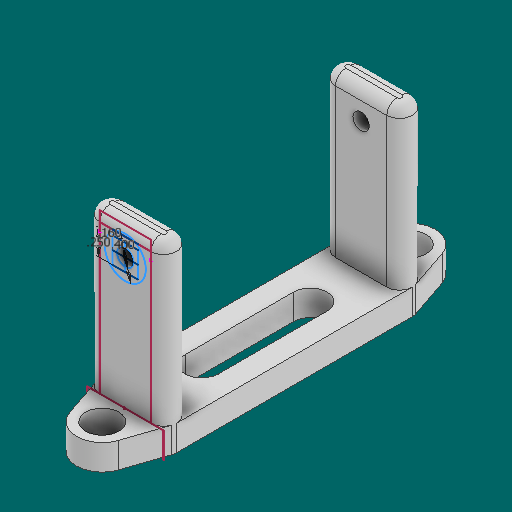
# Autodesk Inventor part: Latest_Odom
Saved by Autodesk Inventor 2025.2 (Build 292293000, 293)
## iProperties
Created: 2024-11-18
Part Number: Latest_Odom
Material: Generic
Document SubType Name: Modeling
Designer: colli
Density: 1 g/cm^3
Appearance: Default
Author: colli
Autodesk Inventor part; units mm, degrees
ref_plane "YZ Plane" through (0, 0, 0) normal (1, 0, 0) x (0, 1, 0)
ref_plane "XZ Plane" through (0, 0, 0) normal (0, 1, 0) x (-1, 0, 0)
ref_plane "XY Plane" through (0, 0, 0) normal (0, 0, 1) x (1, 0, 0)
sketch "Sketch1" plane through (0, 0, 0) normal (0, 1, 0) x (-1, 0, 0)
  line L0 (1.8331, -34.925) -> (-1.8331, -34.925)
  line L1 (-1.8331, -34.925) -> (-3.6662, -31.75)
  line L2 (-3.6662, -31.75) -> (-1.8331, -28.575)
  line L3 (-1.8331, -28.575) -> (1.8331, -28.575)
  line L4 (1.8331, -28.575) -> (3.6662, -31.75)
  line L5 (3.6662, -31.75) -> (1.8331, -34.925)
  circle A0 centre (0, -31.75) radius 2.0955
  circle A1 centre (0, -31.75) radius 3.0353
  line L6 (-31.877, 19.812) -> (-31.877, -7.112)
  line L7 (-31.877, -7.112) -> (31.877, -7.112)
  line L8 (31.877, -7.112) -> (31.877, 19.812)
  line L9 (31.877, 19.812) -> (-31.877, 19.812)
  line L10 (0, 6.35) -> (31.877, 6.35)
  line L11 (0, 6.35) -> (-31.877, 6.35)
  arc A2 (-6.0168, -33.7799) -> (6.0168, -33.7799) centre (0, -31.75) ccw
  line L12 (-6.35, -26.035) -> (6.35, -26.035)
  line L13 (6.35, -19.685) -> (-6.35, -19.685)
  arc A3 (-6.35, -19.685) -> (-6.35, -26.035) centre (-6.35, -22.86) ccw
  arc A4 (6.35, -26.035) -> (6.35, -19.685) centre (6.35, -22.86) ccw
  line L14 (9.525, -22.86) -> (9.525, -7.112)
  line L15 (6.0168, -33.7799) -> (9.3584, -23.8749)
  line L16 (-9.525, -7.112) -> (-9.525, -22.86)
  line L17 (-9.3584, -23.8749) -> (-6.0168, -33.7799)
  line L18 (1.8331, 47.625) -> (-1.8331, 47.625)
  line L19 (-1.8331, 47.625) -> (-3.6662, 44.45)
  line L20 (-3.6662, 44.45) -> (-1.8331, 41.275)
  line L21 (-1.8331, 41.275) -> (1.8331, 41.275)
  line L22 (1.8331, 41.275) -> (3.6662, 44.45)
  line L23 (3.6662, 44.45) -> (1.8331, 47.625)
  circle A5 centre (0, 44.45) radius 2.0955
  circle A6 centre (0, 44.45) radius 3.0353
  arc A7 (6.0168, 46.4799) -> (-6.0168, 46.4799) centre (0, 44.45) ccw
  line L24 (-6.35, 38.735) -> (6.35, 38.735)
  line L25 (6.35, 32.385) -> (-6.35, 32.385)
  arc A8 (-6.35, 38.735) -> (-6.35, 32.385) centre (-6.35, 35.56) ccw
  arc A9 (6.35, 32.385) -> (6.35, 38.735) centre (6.35, 35.56) ccw
  line L26 (6.0168, 46.4799) -> (9.3584, 36.5749)
  line L27 (-9.3584, 36.5749) -> (-6.0168, 46.4799)
  line L28 (9.525, 35.56) -> (9.525, 19.812)
  line L29 (-9.525, 35.56) -> (-9.525, 19.812)
  circle A10 centre (0, 44.45) radius 4.1275
  circle A11 centre (0, -31.75) radius 4.1275
  line L30 (-9.525, 19.812) -> (-9.525, -7.112)
  line L31 (9.525, 19.812) -> (9.525, -7.112)
  line L32 (0, 19.812) -> (0, -7.112) construction
  line L33 (4.1275, 19.812) -> (4.1275, -7.112)
  line L34 (-4.1275, -7.112) -> (-4.1275, 19.812)
  arc A12 (4.1275, 19.812) -> (-4.1275, 19.812) centre (0, 19.812) ccw
  arc A13 (-4.1275, -7.112) -> (4.1275, -7.112) centre (0, -7.112) ccw
  point P0 (0, 0)
  point P1 (0, 6.35)
  dimension "d35" = 8.255
  dimension "d36" = 8.255
  constraints: 72 end point, 22 point on circle, 21 symmetric about line, 15 tangent, 14 centre point, 5 midpoint, 4 coincident, 4 perpendicular, 4 point on line, 3 parallel, 1 horizontal, 1 vertical, 5 other
  measures "d35" diameter of A10
  measures "d36" diameter of A11
extrude "Extrusion1" add sketch "Sketch1" against normal blind 6.35 contours L29 A8 L25 A9 L28 L9 A12 | L9 L34 L11 L30 | L11 L34 L7 L30 | A8 L24 A9 L25 | L7 A13 L14 A4 L13 A3 L16 | L9 L31 L10 L33 | L27 A7 L26 A9 L24 A8 | A3 L13 A4 L12 | L10 L31 L7 L33 | A3 L12 A4 L15 A2 L17
extrude "Extrusion2" add sketch "Sketch1" along normal blind 39.37 contours A8 L24 A9 L25 | A3 L13 A4 L12
fillet "Fillet1" radius 2.54 8 edges at (9.525, 39.37, 35.56) (0, 39.37, 32.385) (-9.525, 39.37, 35.56) (0, 39.37, 38.735) (0, 39.37, -26.035) (-9.525, 39.37, -22.86) (0, 39.37, -19.685) (9.525, 39.37, -22.86)
sketch "Sketch2" plane through (-6.35, 0, 38.735) normal (0, 0, 1) x (1, 0, 0)
  line L0 (0, 0) -> (0, 36.83) projected
  line L1 (12.7, 0) -> (0, 0) projected
  line L2 (12.7, 0) -> (12.7, 36.83) projected
  line L3 (12.7, 36.83) -> (12.7, 39.37) projected
  line L4 (12.7, 36.83) -> (0, 36.83) projected
  line L5 (0, 36.83) -> (0, 39.37) projected
  line L6 (0, 36.83) -> (0, 39.37) projected
  line L7 (0, 36.83) -> (0, 36.83) projected
  line L8 (0, 0) -> (0, 36.83) projected
  line L9 (12.7, 36.83) -> (12.7, 36.83) projected
  line L10 (12.7, 0) -> (12.7, 36.83) projected
  line L11 (15.7084, 0) -> (12.7, 0) projected
  line L12 (15.7084, 0) -> (15.7084, -6.35) projected
  line L13 (15.875, -6.35) -> (15.7084, -6.35) projected
  line L14 (15.875, 0) -> (15.875, -6.35) projected
  line L15 (12.7, 0) -> (15.875, 0) projected
  line L16 (12.7, 0) -> (12.7, 36.83) projected
  line L17 (12.7, 34.925) -> (12.7, 39.37) projected
  line L18 (12.7, 0) -> (12.7, 36.83) projected
  line L19 (12.7, 0) -> (12.7, 36.83) projected
  line L20 (12.7, 36.83) -> (12.7, 39.37) projected
  line L21 (12.7, 36.83) -> (12.7, 36.83) projected
  line L22 (0, 36.83) -> (0, 36.83) projected
  line L23 (0, 0) -> (0, 36.83) projected
  line L24 (-3.175, 0) -> (0, 0) projected
  line L25 (-3.175, 0) -> (-3.175, -6.35) projected
  line L26 (-3.0084, -6.35) -> (-3.175, -6.35) projected
  line L27 (-3.0084, 0) -> (-3.0084, -6.35) projected
  line L28 (0, 0) -> (-3.0084, 0) projected
  line L29 (0, 0) -> (0, 36.83) projected
  line L30 (12.7, 39.37) -> (12.7, 36.83) projected
  line L31 (12.7, 39.37) -> (12.7, 39.37) projected
  line L32 (0, 36.83) -> (0, 39.37) projected
  line L33 (0, 39.37) -> (0, 39.37) projected
  line L34 (0, 39.37) -> (12.7, 39.37) projected
  line L35 (0, 36.83) -> (12.7, 36.83) projected
  line L36 (0, 36.83) -> (12.7, 36.83) projected
  line L37 (6.35, 36.83) -> (3.175, 36.83)
  line L38 (3.175, 29.21) -> (9.525, 29.21)
  line L39 (9.525, 36.83) -> (3.175, 36.83)
  line L40 (3.175, 29.21) -> (3.175, 35.56)
  line L41 (3.175, 35.56) -> (9.525, 35.56)
  line L42 (9.525, 35.56) -> (9.525, 29.21)
  line L43 (6.35, 35.56) -> (6.35, 29.21)
  line L44 (3.175, 32.385) -> (9.525, 32.385)
  circle A0 centre (6.35, 32.385) radius 2.032
  circle A1 centre (6.35, 32.385) radius 5.08
  point P0 (6.35, 0)
  point P1 (0, 34.925)
  point P2 (0, 34.925)
  point P3 (0, 34.925)
  dimension "d43" = 6.35
  dimension "d46" = 4.064
  dimension "d49" = 10.16
  constraints: 16 end point, 4 midpoint, 2 centre point, 2 horizontal, 2 perpendicular, 1 coincident, 1 vertical, 4 other
  measures "d43" distance of L38.start L40.end
  measures "d46" diameter of A0
  measures "d49" diameter of A1
extrude "Extrusion4" cut sketch "Sketch2" along normal through all both and the other way through all contours A0 L44 L43 | L43 L44 A0 | A0 L43 L44 | L43 A0 L44
body "Solid1"
